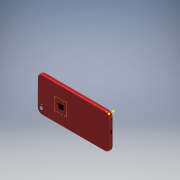
# Autodesk Inventor part: telefon
Saved by Autodesk Inventor 2018 (Build 220112000, 112)
## iProperties
Created: 2018-05-15
Part Number: telefon
Material: Generic
Document SubType Name: Modeling
Designer: dilan haddad
Density: 1 g/cm^3
Appearance: Default
Author: dilan haddad
Autodesk Inventor part; units mm, degrees
ref_plane "YZ Plane" through (0, 0, 0) normal (1, 0, 0) x (0, 1, 0)
ref_plane "XZ Plane" through (0, 0, 0) normal (0, 1, 0) x (-1, 0, 0)
ref_plane "XY Plane" through (0, 0, 0) normal (0, 0, 1) x (1, 0, 0)
sketch "Sketch1" plane through (0, 0, 0) normal (0, 1, 0) x (-1, 0, 0)
  line L0 (0, 0) -> (138, 0)
  line L1 (138, 0) -> (138, -67)
  line L2 (138, -67) -> (0, -67)
  line L3 (0, -67) -> (0, 0)
  dimension "d0" = 138
  dimension "d1" = 67
  constraints: 8 end point, 2 parallel, 1 horizontal, 1 perpendicular
  measures "d0" distance of L1.end L2.end
  measures "d1" distance of L0.end L1.end
extrude "Extrusion1" add sketch "Sketch1" along normal blind 8
fillet "Fillet3" radius 9 4 edges at (-138, 4, 0) (-138, 4, -67) (0, 4, 0) (0, 4, -67)
fillet "Fillet4" radius 2.5 16 edges at (-135.364, 8, -2.636) (-69, 8, 0) (-2.636, 8, -2.636) (0, 8, -33.5) (-2.636, 8, -64.364) (-69, 8, -67) (-135.364, 8, -64.364) (-138, 8, -33.5) (0, 0, -33.5) (-2.636, 0, -64.364) (-69, 0, -67) (-135.364, 0, -64.364) (-138, 0, -33.5) (-135.364, 0, -2.636) (-69, 0, 0) (-2.636, 0, -2.636)
sketch "Sketch9" plane through (0, 8, 0) normal (0, 1, 0) x (1, 0, 0)
  line L0 (-135.5, 9) -> (-135.5, 58) projected
  line L1 (-2.5, 58) -> (-2.5, 9) projected
  line L2 (-9, 2.5) -> (-129, 2.5) projected
  line L3 (-129, 64.5) -> (-9, 64.5) projected
  line L4 (-121, 4.5) -> (-17, 4.5)
  line L5 (-17, 4.5) -> (-17, 62.5)
  line L6 (-17, 62.5) -> (-121, 62.5)
  line L7 (-121, 62.5) -> (-121, 4.5)
  point P0 (0, 0)
  constraints: 8 end point, 2 parallel, 1 horizontal, 1 perpendicular
sketch "Sketch11" plane through (0, 8, 0) normal (0, 1, 0) x (1, 0, 0)
  line L0 (-2.5, 58) -> (-2.5, 9) projected
  circle A0 centre (-9.7532, 33.5) radius 4.75
  line L1 (-135.5, 9) -> (-135.5, 58) projected
  circle A1 centre (-133.0353, 33.5) radius 0.5
  line L2 (-129.849, 33.5) -> (-129.849, 38)
  line L3 (-129.849, 38) -> (-130.449, 38)
  line L4 (-130.449, 38) -> (-130.449, 33.5)
  line L5 (-130.449, 33.5) -> (-130.449, 29)
  line L6 (-130.449, 29) -> (-129.849, 29)
  line L7 (-129.849, 29) -> (-129.849, 33.5)
  circle A2 centre (-130.149, 27.1522) radius 0.5173
  line L8 (-130.449, 29) -> (-129.849, 29)
  line L9 (-129.849, 29) -> (-129.849, 38)
  line L10 (-129.849, 38) -> (-130.449, 38)
  line L11 (-130.449, 38) -> (-130.449, 29)
  point P0 (0, 0)
  dimension "d21" = 9.5
  dimension "d22" = 1
  constraints: 20 end point, 4 parallel, 3 centre point, 1 horizontal, 1 perpendicular, 1 point on line
  measures "d21" diameter of A0
  measures "d22" diameter of A1
extrude "Extrusion2" cut sketch "Sketch11" against normal blind 0.3
sketch "Sketch12" plane through (0, 8, 0) normal (0, 1, 0) x (1, 0, 0)
  line L0 (-121.0067, 4.7801) -> (-121.0067, 62.5653) construction
  line L1 (-121.0067, 62.5653) -> (-18.2774, 62.5653) construction
  line L2 (-18.2774, 62.5653) -> (-18.2774, 4.7801) construction
  line L3 (-18.2774, 4.7801) -> (-121.0067, 4.7801) construction
  point P0 (0, 0)
  constraints: 2 other
sketch "Sketch15" plane through (0, 2.5, -58) normal (1, 0, 0) x (0, 0, -1)
  line L0 (-49, 0) -> (-49, 3) projected
  line L1 (0, 3) -> (0, 0) projected
  circle A0 centre (-3.6879, 1.5) radius 0.7
  circle A1 centre (-5.8468, 1.5) radius 0.7
  circle A2 centre (-8.0674, 1.5) radius 0.7
  circle A3 centre (-10.3497, 1.5) radius 0.7
  circle A4 centre (-12.5703, 1.5) radius 0.7
  point P0 (-58, -2.5)
  constraints: 5 centre point
extrude "Extrusion5" cut sketch "Sketch15" against normal blind 0.6
sketch "Sketch16" plane through (0, 2.5, -58) normal (1, 0, 0) x (0, 0, -1)
  point P0 (-58, -2.5)
sketch "Sketch17" plane through (0, 2.5, -58) normal (1, 0, 0) x (0, 0, -1)
  line L0 (-49, 0) -> (-49, 3) projected
  line L1 (-49, 1.5) -> (0, 1.5)
  line L2 (0, 3) -> (0, 0) projected
  line L3 (-49, 3) -> (0, 3) projected
  line L4 (-24.5, 3) -> (-24.5, 0)
  circle A0 centre (-46.1363, 1.5) radius 1.15
  line L5 (-27.6835, 2.2868) -> (-21.9014, 2.2868)
  line L6 (-21.2014, 1.5868) -> (-21.2014, 1.4809)
  line L7 (-21.9014, 0.7809) -> (-27.6835, 0.7809)
  line L8 (-28.3835, 1.4809) -> (-28.3835, 1.5868)
  arc A1 (-27.6835, 2.2868) -> (-28.3835, 1.5868) centre (-27.6835, 1.5868) ccw
  arc A2 (-28.3835, 1.4809) -> (-27.6835, 0.7809) centre (-27.6835, 1.4809) ccw
  arc A3 (-21.2014, 1.5868) -> (-21.9014, 2.2868) centre (-21.9014, 1.5868) ccw
  arc A4 (-21.9014, 0.7809) -> (-21.2014, 1.4809) centre (-21.9014, 1.4809) ccw
  point P0 (-58, -2.5)
  dimension "d67" = 0.7
  dimension "d68" = 0.7
  constraints: 12 end point, 8 point on circle, 8 tangent, 5 centre point, 3 midpoint, 2 equal radius, 2 parallel, 1 horizontal, 1 perpendicular, 1 point on line, 1 vertical
  measures "d67" radius of A1
  measures "d68" radius of A3
extrude "Extrusion6" cut sketch "Sketch17" against normal blind 4 contours A0 L1 | L1 A0 | L5 A3 L6 L1 L4 | L4 L1 L8 A1 L5 | L1 L4 L7 A2 L8 | L1 L6 A4 L7 L4
sketch "Sketch18" plane through (-129, 2.5, 0) normal (0, 0, 1) x (1, 0, 0)
  line L0 (0, 0) -> (0, 3) projected
  line L1 (0, 1.5) -> (120, 1.5)
  line L2 (120, 0) -> (129, 0) projected
  line L3 (17.633, 1.989) -> (25.3803, 1.989)
  line L4 (25.8803, 1.489) -> (25.8803, 1.2394)
  line L5 (25.3803, 0.7394) -> (17.633, 0.7394)
  line L6 (17.133, 1.2394) -> (17.133, 1.489)
  line L7 (29.1572, 1.989) -> (36.4879, 1.989)
  line L8 (36.9879, 1.489) -> (36.9879, 1.2394)
  line L9 (36.4879, 0.7394) -> (29.1572, 0.7394)
  line L10 (28.6572, 1.2394) -> (28.6572, 1.489)
  arc A0 (17.633, 1.989) -> (17.133, 1.489) centre (17.633, 1.489) ccw
  arc A1 (17.133, 1.2394) -> (17.633, 0.7394) centre (17.633, 1.2394) ccw
  arc A2 (25.8803, 1.489) -> (25.3803, 1.989) centre (25.3803, 1.489) ccw
  arc A3 (25.3803, 0.7394) -> (25.8803, 1.2394) centre (25.3803, 1.2394) ccw
  arc A4 (29.1572, 1.989) -> (28.6572, 1.489) centre (29.1572, 1.489) ccw
  arc A5 (28.6572, 1.2394) -> (29.1572, 0.7394) centre (29.1572, 1.2394) ccw
  arc A6 (36.9879, 1.489) -> (36.4879, 1.989) centre (36.4879, 1.489) ccw
  arc A7 (36.4879, 0.7394) -> (36.9879, 1.2394) centre (36.4879, 1.2394) ccw
  point P0 (129, -2.5)
  point P1 (28.6572, 1.989)
  point P2 (36.9879, 0.7394)
  dimension "d71" = 0.5
  constraints: 18 end point, 16 point on circle, 16 tangent, 8 centre point, 7 equal radius, 6 point on line, 5 parallel, 2 horizontal, 2 perpendicular, 1 midpoint
  measures "d71" radius of A0
extrude "Extrusion7" add sketch "Sketch18" along normal blind 0.5
sketch "Sketch19" plane through (-129, 2.5, 0) normal (0, 0, 1) x (1, 0, 0)
  line L0 (12.7221, 0.7394) -> (8.2034, 0.7394)
  line L1 (7.9034, 1.0394) -> (7.9034, 1.6002)
  line L2 (8.2034, 1.9002) -> (12.7221, 1.9002)
  line L3 (13.0221, 1.6002) -> (13.0221, 1.0394)
  arc A0 (8.2034, 1.9002) -> (7.9034, 1.6002) centre (8.2034, 1.6002) ccw
  arc A1 (7.9034, 1.0394) -> (8.2034, 0.7394) centre (8.2034, 1.0394) ccw
  arc A2 (13.0221, 1.6002) -> (12.7221, 1.9002) centre (12.7221, 1.6002) ccw
  arc A3 (12.7221, 0.7394) -> (13.0221, 1.0394) centre (12.7221, 1.0394) ccw
  point P0 (129, -2.5)
  dimension "d74" = 0.3
  constraints: 8 end point, 8 point on circle, 8 tangent, 4 centre point, 3 equal radius, 2 parallel, 1 horizontal, 1 perpendicular
  measures "d74" radius of A0
extrude "Extrusion8" cut sketch "Sketch19" against normal blind 0.7
sketch "Sketch20" plane through (-129, 2.5, -0.7) normal (0, 0, 1) x (1, 0, 0)
  line L0 (12.7071, 1.7577) -> (8.1711, 1.7577)
  line L1 (8.0711, 1.6577) -> (8.0711, 1.5231)
  line L2 (8.1711, 1.4231) -> (12.7071, 1.4231)
  line L3 (12.8071, 1.5231) -> (12.8071, 1.6577)
  arc A0 (12.8071, 1.6577) -> (12.7071, 1.7577) centre (12.7071, 1.6577) ccw
  arc A1 (12.7071, 1.4231) -> (12.8071, 1.5231) centre (12.7071, 1.5231) ccw
  arc A2 (8.1711, 1.7577) -> (8.0711, 1.6577) centre (8.1711, 1.6577) ccw
  arc A3 (8.0711, 1.5231) -> (8.1711, 1.4231) centre (8.1711, 1.5231) ccw
  point P0 (129, -2.5)
  dimension "d77" = 0.1
  dimension "d78" = 0.1
  constraints: 8 end point, 8 point on circle, 8 tangent, 4 centre point, 2 equal radius, 2 parallel, 1 horizontal, 1 perpendicular
  measures "d77" radius of A0
  measures "d78" radius of A2
extrude "Extrusion9" add sketch "Sketch20" along normal blind 0.9
sketch "Sketch21" plane through (-9, 2.5, -67) normal (0, 0, -1) x (-1, 0, 0)
  line L0 (107.2779, 0.7394) -> (111.7966, 0.7394) projected
  line L1 (102.367, 1.989) -> (94.6197, 1.989) projected
  line L2 (109.0372, 0.7394) -> (102.3642, 0.7394)
  line L3 (101.8642, 1.2394) -> (101.8642, 1.489)
  line L4 (102.3642, 1.989) -> (109.0372, 1.989)
  line L5 (109.5372, 1.489) -> (109.5372, 1.2394)
  arc A0 (101.8642, 1.2394) -> (102.3642, 0.7394) centre (102.3642, 1.2394) ccw
  arc A1 (102.3642, 1.989) -> (101.8642, 1.489) centre (102.3642, 1.489) ccw
  arc A2 (109.0372, 0.7394) -> (109.5372, 1.2394) centre (109.0372, 1.2394) ccw
  arc A3 (109.5372, 1.489) -> (109.0372, 1.989) centre (109.0372, 1.489) ccw
  point P0 (-9, -2.5)
  point P1 (109.5372, 0.7394)
  point P2 (101.8642, 1.989)
  dimension "d81" = 0.5
  constraints: 8 end point, 8 point on circle, 8 tangent, 5 point on line, 4 centre point, 3 equal radius, 2 parallel, 1 horizontal, 1 midpoint, 1 perpendicular
  measures "d81" radius of A0
extrude "Extrusion10" add sketch "Sketch21" along normal blind 0.5
sketch "Sketch22" plane through (0, 0, 0) normal (0, -1, 0) x (1, 0, 0)
  point P0 (0, 0)
sketch "Sketch23" plane through (0, 0, 0) normal (0, -1, 0) x (1, 0, 0)
  circle A0 centre (-128.9815, -54.6956) radius 3.03
  circle A1 centre (-128.9815, -48.6898) radius 1.1168
  point P0 (0, 0)
  constraints: 2 centre point
extrude "Extrusion11" add sketch "Sketch23" along normal blind 1 contours A0
sketch "Sketch24" plane through (-128.9815, -1, -54.6956) normal (0, -1, 0) x (1, 0, 0)
  circle A0 centre (0, 0) radius 2.5382
  point P0 (128.9815, 54.6956)
  constraints: 1 centre point
extrude "Extrusion12" cut sketch "Sketch24" against normal blind 0.3
sketch "Sketch25" plane through (-128.9815, -0.7, -54.6956) normal (0, -1, 0) x (1, 0, 0)
  circle A0 centre (0, 0) radius 1.6518
  point P0 (128.9815, 54.6956)
  constraints: 1 centre point
extrude "Extrusion13" add sketch "Sketch25" along normal blind 0.3
sketch "Sketch26" plane through (-128.9815, -1, -54.6956) normal (0, -1, 0) x (1, 0, 0)
  circle A0 centre (0, 0) radius 0.4872
  point P0 (128.9815, 54.6956)
  constraints: 1 centre point
extrude "Extrusion14" cut sketch "Sketch26" against normal blind 0.3
sketch "Sketch27" plane through (0, 0, 0) normal (0, -1, 0) x (1, 0, 0)
  circle A0 centre (-128.9815, -49.2163) radius 0.9142
  point P0 (0, 0)
  constraints: 1 centre point
extrude "Extrusion15" cut sketch "Sketch27" against normal blind 0.3
sketch "Sketch28" plane through (0, 0, 0) normal (0, -1, 0) x (1, 0, 0)
  line L0 (-105.2991, -46.5746) -> (-105.2991, -22.5188) construction
  line L1 (-105.2991, -22.5188) -> (-81.2433, -22.5188) construction
  line L2 (-81.2433, -22.5188) -> (-81.2433, -46.5746) construction
  line L3 (-81.2433, -46.5746) -> (-105.2991, -46.5746) construction
  point P0 (0, 0)
  constraints: 2 other
body "Solid1"
